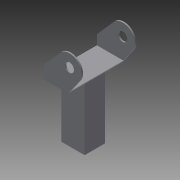
# Autodesk Inventor part: Elbow_Pitch
Saved by Autodesk Inventor 2013 (Build 170138000, 138)
## iProperties
Created: 2012-12-04
Part Number: Elbow_Pitch
Material: Generic
Document SubType Name: Modeling
Designer: Joe
Density: 1 g/cm^3
Author: Joe
Autodesk Inventor part; units mm, degrees
ref_plane "YZ Plane" through (0, 0, 0) normal (1, 0, 0) x (0, 1, 0)
ref_plane "XZ Plane" through (0, 0, 0) normal (0, 1, 0) x (-1, 0, 0)
ref_plane "XY Plane" through (0, 0, 0) normal (0, 0, 1) x (1, 0, 0)
sketch "Sketch1" plane through (0, 0, 0) normal (1, 0, 0) x (0, 1, 0)
  circle A0 centre (0, 0) radius 10
  line L0 (0, 0) -> (-50.6762, -56.6385) construction
  line L1 (-50.6762, -56.6385) -> (-50.6762, -2.6385)
  line L2 (-50.6762, -56.6385) -> (-23.6762, -56.6385)
  arc A1 (17.7921, -20.3086) -> (-15.5352, 22.083) centre (0, 0) ccw
  line L3 (-50.6762, -2.6385) -> (-15.5352, 22.083)
  line L4 (-23.6762, -56.6385) -> (17.7921, -20.3086)
  dimension "d0" = 20
  dimension "d2" = 41.82
  dimension "d5" = 76
  dimension "d6" = 27
  dimension "d7" = 54
  dimension "d8" = 54
  constraints: 10 end point, 2 centre point, 2 coincident, 2 point on circle, 2 tangent, 1 perpendicular, 1 vertical
  measures "d0" diameter of A0
  measures "d2" angle of L0 L1
  measures "d5" distance of L0.start L0.end
  measures "d6" distance of L0.end L2.end
  measures "d7" distance of L0.end L1.end
  measures "d8" diameter of A1
extrude "Extrusion1" add sketch "Sketch1" along normal mid plane 120
sketch "Sketch2" plane through (0, 0, 0) normal (1, 0, 0) x (0, 1, 0)
  circle A0 centre (0, 0) radius 10 projected
  line L0 (-50.6762, -2.6385) -> (-50.6762, -56.6385) projected
  line L1 (-50.6762, -56.6385) -> (-23.6762, -56.6385) projected
  line L2 (-23.6762, -56.6385) -> (17.7921, -20.3086) projected
  arc A1 (17.7921, -20.3086) -> (-15.5352, 22.083) centre (0, 0) ccw projected
  line L3 (-15.5352, 22.083) -> (-50.6762, -2.6385) projected
  line L4 (-44.6762, -56.6385) -> (-44.6762, 1.5825)
  line L5 (-44.6762, 1.5825) -> (-15.5352, 22.083)
  line L6 (-44.6762, -56.6385) -> (-23.6762, -56.6385)
  dimension "d11" = 6
  constraints: 6 end point, 2 perpendicular, 2 point on line
  measures "d11" distance between parallel lines of L0 L4
extrude "Extrusion2" cut sketch "Sketch2" along normal mid plane 114 contours L3 A1 L2 L1 L4
sketch "Sketch3" plane through (0, 0, 0) normal (1, 0, 0) x (0, 1, 0)
  line L0 (-50.6762, -29.6385) -> (-80.5956, -29.6385) construction
  line L1 (-50.6762, -2.6385) -> (-50.6762, -56.6385) projected
  line L2 (-50.6762, -4.1385) -> (-187.6762, -4.1385)
  line L3 (-187.6762, -4.1385) -> (-187.6762, -55.1385)
  line L4 (-187.6762, -55.1385) -> (-50.6762, -55.1385)
  line L5 (-50.6762, -55.1385) -> (-50.6762, -4.1385)
  line L6 (-50.6762, -29.6385) -> (-187.6762, -29.6385) construction
  point P0 (0, 0)
  dimension "d14" = 51
  dimension "d16" = 137
  constraints: 12 end point, 6 midpoint, 2 collinear, 2 horizontal, 2 parallel, 1 perpendicular, 1 point on line
  measures "d14" distance of L2.end L3.end
  measures "d16" distance of L3.end L4.end
extrude "Extrusion3" add sketch "Sketch3" along normal mid plane 45
sketch "Sketch5" plane through (-22.5, -187.6762, -55.1385) normal (0, -1, 0) x (1, 0, 0)
  line L0 (0, 51) -> (45, 0) construction
  circle A0 centre (22.5, 25.5) radius 10
  point P0 (22.5, 55.1385)
  dimension "d19" = 20
  constraints: 2 end point, 1 centre point, 1 midpoint
  measures "d19" diameter of A0
extrude "Extrusion4" cut sketch "Sketch5" against normal blind 10
move or copy body "Move Body6" bodies to move or copy 1 copy no rotation origin (0, 0, 0) rotation axis (1, 0, 0) rotation angle 90
move or copy body "Move Body7" bodies to move or copy 1 copy no rotation origin (0, 0, 0) rotation axis (0, 0, 1) rotation angle 90
body "Solid1"
